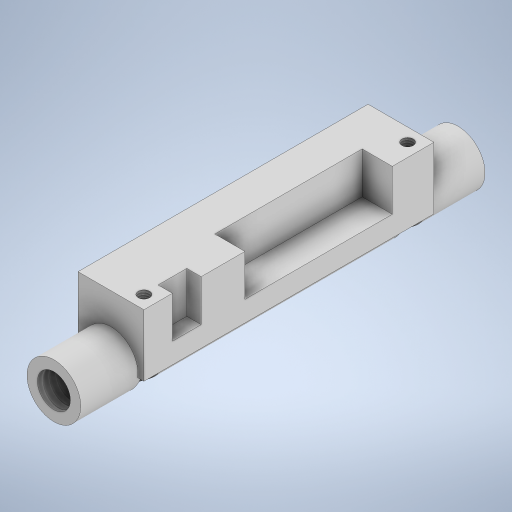
# Autodesk Inventor part: Line Sensor 6 Bracket
Saved by Autodesk Inventor 2024 (Build 280153000, 153)
## iProperties
Created: 2023-10-20
Part Number: Line Sensor 6 Bracket
Material: Generic
Document SubType Name: Modeling
Designer: olson
Density: 1 g/cm^3
Appearance: Default
Author: olson
Autodesk Inventor part; units mm, degrees
ref_plane "YZ Plane" through (0, 0, 0) normal (1, 0, 0) x (0, 1, 0)
ref_plane "XZ Plane" through (0, 0, 0) normal (0, 1, 0) x (-1, 0, 0)
ref_plane "XY Plane" through (0, 0, 0) normal (0, 0, 1) x (1, 0, 0)
sketch "Sketch1" plane through (0, 0, 0) normal (0, 1, 0) x (-1, 0, 0)
  line L0 (0, -55.88) -> (-12.7, -55.88)
  line L1 (-12.7, 0) -> (0, 0)
  line L2 (0, 0) -> (0, -20.94)
  line L3 (0, -34.94) -> (0, -55.88)
  line L4 (-12.7, -55.88) -> (-12.7, -34.94)
  line L5 (-12.7, -20.94) -> (-12.7, 0)
  line L6 (0, -20.94) -> (0, -34.94)
  line L7 (-12.7, -20.94) -> (-12.7, -34.94)
  dimension "d1" = 55.88
  dimension "d2" = 12.7
  constraints: 16 end point, 4 perpendicular, 2 collinear, 2 vertical, 1 horizontal
  measures "d1" distance of L1.end L0.start
  measures "d2" distance of L0.start L0.end
extrude "Extrusion1" add sketch "Sketch1" along normal blind 1.5
sketch "Sketch2" plane through (0, 1.5, 0) normal (0, 1, 0) x (1, 0, 0)
  line L0 (12.7, 0) -> (12.7, 55.88) projected
  line L1 (12.7, 0) -> (10.16, 0)
  line L2 (12.7, 2.54) -> (12.7, 0)
  circle A0 centre (10.16, 2.54) radius 1.092
  circle A1 centre (10.16, 53.34) radius 1.092
  point P0 (0, 0)
  dimension "d8" = 2.184
  dimension "d10" = 2.184
  constraints: 4 end point, 2 centre point, 1 horizontal
  measures "d8" diameter of A0
  measures "d10" diameter of A1
extrude "Extrusion2" cut sketch "Sketch2" against normal blind 1.5
sketch "Sketch5" plane through (0, 0, 0) normal (0, 0, 1) x (1, 0, 0)
  line L0 (12.7, 0) -> (0, 0) projected
  line L1 (6.35, 0) -> (6.35, 1.5)
  line L2 (12.7, 1.5) -> (0, 1.5) projected
  line L3 (0, 0) -> (0, 1.5) projected
  line L4 (0, 0.75) -> (12.7, 0.75)
  line L5 (12.7, 0) -> (12.7, 1.5) projected
  circle A0 centre (6.35, 0.75) radius 5.175
  dimension "d30" = 10.35
  constraints: 4 end point, 4 midpoint, 1 centre point
  measures "d30" diameter of A0
extrude "Extrusion5" add sketch "Sketch5" along normal blind 2 contours A0 L0 | L0 L1 L4 A0 | L0 A0 L4 L1 | L4 L1 L2 A0 | L4 A0 L2 L1 | L2 A0
sketch "Sketch6" plane through (6.35, 0.75, 2) normal (0, 0, 1) x (1, 0, 0)
  circle A0 centre (0, 0) radius 5.175
  circle A1 centre (0, 0) radius 3.175
  point P0 (-6.35, -0.75)
  dimension "d35" = 6.35
  constraints: 2 centre point, 1 coincident
  measures "d35" diameter of A1
extrude "Extrusion6" add sketch "Sketch6" along normal blind 9
sketch "Sketch7" plane through (12.7, 0, -55.88) normal (0, 0, -1) x (-1, 0, 0)
  line L0 (0, 0) -> (0, 1.5) projected
  line L1 (0, 0.75) -> (12.7, 0.75)
  line L2 (12.7, 0) -> (12.7, 1.5) projected
  line L3 (11.4704, 1.5) -> (1.2296, 1.5) projected
  line L4 (6.35, 1.5) -> (6.35, 0)
  circle A0 centre (6.35, 0.75) radius 5.175
  constraints: 4 end point, 4 midpoint, 1 centre point, 1 perpendicular
extrude "Extrusion7" add sketch "Sketch7" along normal blind 2
sketch "Sketch8" plane through (6.35, 0.75, -57.88) normal (0, 0, -1) x (-1, 0, 0)
  circle A0 centre (0, 0) radius 5.175
  circle A1 centre (0, 0) radius 3.175
  point P0 (6.35, -0.75)
  dimension "d40" = 6.35
  constraints: 2 centre point, 1 coincident
  measures "d40" diameter of A1
extrude "Extrusion8" add sketch "Sketch8" along normal blind 9
thread "Thread1" size "1/4-20 UNC" class "2B" standard "ANSI Unified Screw Threads" full length
thread "Thread2" size "1/4-20 UNC" class "2B" standard "ANSI Unified Screw Threads" full length
sketch "Sketch9" plane through (0, 0, 0) normal (0, 0, -1) x (-1, 0, 0)
  arc A0 (-11.4704, 0) -> (-1.2296, 0) centre (-6.35, 0.75) ccw projected
  line L0 (0, 0) -> (-1.2296, 0) projected
  line L1 (-11.4704, 0) -> (-1.2296, 0)
  circle A1 centre (-6.35, 0.75) radius 5.175
  constraints: 2 end point, 1 centre point, 1 coincident, 1 concentric, 1 horizontal
extrude "Extrusion9" add sketch "Sketch9" along normal up to next contours L1 A0
sketch "Sketch10" plane through (10.16, 0, -2.54) normal (0, 1, 0) x (1, 0, 0)
  circle A0 centre (0, 0) radius 1.092
  circle A1 centre (0, 50.8) radius 1.092 projected
  circle A2 centre (0, 50.8) radius 1.092
  point P0 (-10.16, -2.54)
  dimension "d60" = 2.184
  constraints: 2 centre point, 1 coincident
  measures "d60" diameter of A0
extrude "Extrusion10" cut sketch "Sketch10" against normal up to next
sketch "Sketch12" plane through (0, 1.5, 0) normal (0, 1, 0) x (1, 0, 0)
  circle A0 centre (10.16, 2.54) radius 1.092 projected
  circle A1 centre (10.16, 2.54) radius 1.092
  circle A2 centre (10.16, 2.54) radius 2.2225
  circle A3 centre (10.16, 53.34) radius 1.092 projected
  circle A4 centre (10.16, 53.34) radius 1.092
  circle A5 centre (10.16, 53.34) radius 2.2225
  point P0 (0, 0)
  dimension "d54" = 4.445
  dimension "d55" = 4.445
  constraints: 4 centre point, 4 coincident
  measures "d54" diameter of A2
  measures "d55" diameter of A5
extrude "Extrusion11" cut sketch "Sketch12" against normal blind 5.925
sketch "Sketch13" plane through (0, 1.5, 0) normal (0, 1, 0) x (1, 0, 0)
  line L0 (12.7, 0) -> (12.7, 55.88) projected
  line L1 (12.7, 55.88) -> (0, 55.88)
  line L2 (0, 55.88) -> (0, 0)
  line L3 (0, 0) -> (12.7, 0)
  line L4 (12.7, 0) -> (12.7, 55.88)
  circle A0 centre (10.16, 53.34) radius 1.092 projected
  circle A1 centre (10.16, 53.34) radius 1.092
  circle A2 centre (10.16, 2.54) radius 1.092 projected
  circle A3 centre (10.16, 2.54) radius 1.092
  constraints: 8 end point, 2 centre point, 2 coincident, 2 parallel, 1 horizontal, 1 perpendicular
extrude "Extrusion12" add sketch "Sketch13" along normal blind 10.4375
thread "Thread5" size "2-56 UNC" class "2B" standard "ANSI Unified Screw Threads" full length
thread "Thread6" size "2-56 UNC" class "2B" standard "ANSI Unified Screw Threads" full length
sketch "Sketch14" plane through (10.16, 1.5, -53.34) normal (0, -1, 0) x (1, 0, 0)
  circle A0 centre (0, 0) radius 1.092 projected
  circle A1 centre (0, 0) radius 2.2225
  circle A2 centre (0, 50.8) radius 2.2225 projected
  circle A3 centre (0, 50.8) radius 2.2225
  circle A4 centre (0, 0) radius 1.092
  circle A5 centre (0, 50.8) radius 1.092
  point P0 (-10.16, 53.34)
  constraints: 4 centre point, 4 coincident, 1 concentric
extrude "Extrusion13" cut sketch "Sketch14" against normal blind 1
sketch "Sketch15" plane through (0, 11.9375, 0) normal (0, 1, 0) x (1, 0, 0)
  line L0 (12.7, 0) -> (12.7, 6.985)
  line L1 (12.7, 0) -> (12.7, 55.88) projected
  line L2 (12.7, 0) -> (19.685, 0) construction
  line L3 (11.525, -11) -> (11.525, 66.88) projected
  line L4 (11.43, 6.985) -> (13.97, 6.985) construction
  line L5 (11.43, 6.985) -> (12.43, 6.985) construction
  line L6 (11.43, 9.525) -> (12.43, 9.525) construction
  line L7 (12.7, 5.985) -> (12.7, 10.525)
  line L8 (12.7, 5.985) -> (12.7, 5.485)
  line L9 (12.7, 5.485) -> (9.93, 5.485)
  line L10 (9.93, 5.485) -> (9.93, 11.025)
  line L11 (9.93, 11.025) -> (12.7, 11.025)
  line L12 (12.7, 11.025) -> (12.7, 10.525)
  point P0 (0, 0)
  dimension "d72" = 90
  dimension "d130" = 0.5
  dimension "d131" = 2.77
  dimension "d132" = 5.54
  constraints: 22 end point, 4 horizontal, 3 perpendicular, 3 point on line, 2 collinear, 1 vertical
  measures "d72" angle of L2 L0
  measures "d130" distance of L7.start L8.end
  measures "d131" distance of L8.end L9.end
  measures "d132" distance of L9.end L10.end
extrude "Extrusion14" cut sketch "Sketch15" against normal blind 8
sketch "Sketch16" plane through (0, 11.9375, 0) normal (0, 1, 0) x (1, 0, 0)
  line L0 (12.7, 0) -> (12.7, 55.88) projected
  line L1 (12.7, 40.234) -> (13.97, 40.234) construction
  line L2 (0, 0) -> (12.7, 0) projected
  line L3 (11.43, 0) -> (40.005, 0) construction
  line L4 (11.525, -11) -> (11.525, 66.88) projected
  line L5 (11.43, 28.575) -> (13.97, 28.575) construction
  line L6 (11.43, 46.355) -> (12.43, 46.355) construction
  line L7 (11.43, 28.575) -> (13.97, 28.575) construction
  line L8 (11.43, 20.955) -> (12.43, 20.955) construction
  line L9 (6.89, 19.955) -> (6.89, 47.355)
  line L10 (12.7, 47.355) -> (12.7, 19.955)
  line L11 (6.89, 47.355) -> (6.89, 47.855)
  line L12 (6.89, 47.855) -> (12.7, 47.855)
  line L13 (12.7, 47.855) -> (12.7, 47.355)
  line L14 (12.7, 19.955) -> (12.7, 19.455)
  line L15 (12.7, 0) -> (12.7, 55.88) projected
  line L16 (12.7, 19.455) -> (6.89, 19.455)
  line L17 (6.89, 19.455) -> (6.89, 19.955)
  point P0 (12.7, 10.525)
  dimension "d123" = 5.81
  dimension "d129" = 28.4
  constraints: 28 end point, 7 point on line, 6 horizontal, 4 perpendicular, 1 collinear, 1 vertical
  measures "d123" distance of L10.end L9.start
  measures "d129" distance between parallel lines of L12 L16
extrude "Extrusion15" cut sketch "Sketch16" against normal blind 8 contours L16 L4 L12 L0 | L16 L17 L9 L11 L12 L4
body "Solid1"
